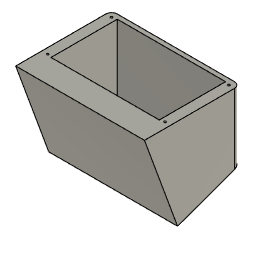
ACInfinityControllerHousing v3 (Autodesk Fusion 360 design; units mm, degrees)
Autodesk Fusion 360 part; units mm, degrees
sketch "Sketch1" plane through (0, 0, 0) normal (0, 0, 1) x (1, 0, 0)
  line L0 (0, 0) -> (113.5, 0)
  line L1 (113.5, 0) -> (113.5, 69.5)
  line L2 (113.5, 69.5) -> (0, 69.5)
  line L3 (0, 69.5) -> (0, 0)
  line L4 (56.75, 69.5) -> (56.75, 0) construction
  line L5 (0, 34.75) -> (113.5, 34.75) construction
  line L6 (-10.75, 74.2) -> (124.25, 74.2)
  line L7 (124.25, 74.2) -> (124.25, -4.7)
  line L8 (124.25, -4.7) -> (-10.75, -4.7)
  line L9 (-10.75, -4.7) -> (-10.75, 74.2)
  line L10 (56.75, 74.2) -> (56.75, -4.7) construction
  line L11 (-10.75, 34.75) -> (124.25, 34.75) construction
  circle A0 centre (-4.75, 68.2) radius 1.1
  circle A1 centre (-4.75, 1.3) radius 1.1
  circle A2 centre (118.25, 1.3) radius 1.1
  circle A3 centre (118.25, 68.2) radius 1.1
  dimension "d1" = 113.5
  dimension "d2" = 69.5
  dimension "d3" = 78.9
  dimension "d4" = 135
  dimension "d5" = 2.2
  dimension "d6" = 2.2
  dimension "d7" = 2.2
  dimension "d8" = 2.2
  dimension "d9" = 6
  dimension "d10" = 6
  dimension "d11" = 6
  dimension "d12" = 6
  dimension "d13" = 6
  dimension "d14" = 6
  dimension "d15" = 6
  dimension "d16" = 6
  constraint horizontal L0
  constraint vertical L1
  constraint horizontal L2
  constraint vertical L3
  constraint coincident L0.start L3.end
  constraint midpoint L2 L4.start
  constraint midpoint L0 L4.end
  constraint midpoint L3 L5.start
  constraint midpoint L1 L5.end
  constraint horizontal L6
  constraint vertical L7
  constraint horizontal L8
  constraint vertical L9
  constraint midpoint L6 L10.start
  constraint midpoint L8 L10.end
  constraint midpoint L9 L11.start
  constraint midpoint L7 L11.end
  constraint collinear L4 L10
  constraint collinear L5 L11
  measures "d1" distance of L0.start L0.end
  measures "d2" distance of L0.start L2.end
  measures "d3" distance of L6.start L8.end
  measures "d4" distance of L7.end L8.end
  measures "d5" diameter of A0
  measures "d6" diameter of A1
  measures "d7" diameter of A2
  measures "d8" diameter of A3
  measures "d9" distance of L6 A0.centre
  measures "d10" distance of L9 A0.centre
  measures "d11" distance of L9 A1.centre
  measures "d12" distance of L8 A1.centre
  measures "d13" distance of L8 A2.centre
  measures "d14" distance of L7 A2.centre
  measures "d15" distance of L7 A3.centre
  measures "d16" distance of L6 A3.centre
extrude "Extrude1" add sketch "Sketch1" against normal blind 30 contours L6 L7 L8 L9 | A0 | A1 | A2 | A3
sketch "Sketch2" plane through (124.25, 0, 0) normal (1, 0, 0) x (0, 1, 0)
  line L0 (74.2, 0) -> (-4.7, 0)
  line L1 (-4.7, 0) -> (-4.7, -30)
  line L2 (-4.7, -30) -> (74.2, -30)
  line L3 (74.2, -30) -> (74.2, 0)
  line L4 (-26.2609, 0) -> (74.2, 0)
  line L5 (-26.2609, 0) -> (8.4215, -95.2891)
  line L6 (8.4215, -95.2891) -> (74.2, -71.3477)
  line L7 (74.2, -71.3477) -> (74.2, 0)
  line L8 (-15.6191, 0) -> (17.8184, -91.8689)
  line L9 (-4.7, 0) -> (-4.7, -30)
  line L10 (69.5, 0) -> (69.5, -73.0584)
  point P0 (69.5, -30)
  point P1 (0, -30)
  dimension "d19" = 70
  dimension "d20" = 10
  dimension "d21" = 70
  dimension "d22" = 90
  constraint coincident L0.start L3.end
  constraint perpendicular L3 L4
  constraint perpendicular L4 L7
  constraint coincident L4 L8.start
  constraint coincident L6 L8.end
  constraint perpendicular L6 L8
  constraint coincident L0.end L1.start
  constraint coincident L1.end L2.start
  constraint coincident L8 L1.end
  constraint coincident L4 L10.start
  constraint coincident L6 L10.end
  constraint perpendicular L4 L10
  constraint coincident P0 L10
  measures "d19" angle of L4 L5
  measures "d20" distance of L1.end L5
  measures "d21" distance of L5.end L6.end
  measures "d22" angle of L5 L6
extrude "Extrude2" add sketch "Sketch2" against normal blind 135 contours L2 L6 L7 L10 | L1 L4 L8 L9 | L4 L5 L6 L8
extrude "Extrude3" add sketch "Sketch2" against normal blind 10.75 contours L2 L6 L8 L10
extrude "Extrude4" add sketch "Sketch2" along normal blind 10.75 from surface at -135 contours L2 L6 L8 L10
chamfer "Chamfer1" distance 4.7 angle 45 1 edges at (56.75, -4.7, -30)
extrude "Extrude5" cut sketch "Sketch1" against normal blind 10 contours A0 | A1 | A2 | A3
fillet "Fillet1" radius 6 2 edges at (124.25, 74.2, -35.6739) (-10.75, 74.2, -35.6739)
